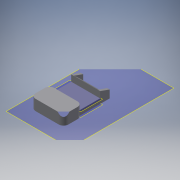
# Autodesk Inventor part: schnapper
Saved by Autodesk Inventor 2016 (Build 200138000, 138)
## iProperties
Created: 2016-06-09
Part Number: schnapper
Material: Generic
Document SubType Name: Modeling
Designer: Chris
Density: 1 g/cm^3
Appearance: Default
Author: Chris
Autodesk Inventor part; units mm, degrees
ref_plane "YZ Plane" through (0, 0, 0) normal (1, 0, 0) x (0, 1, 0)
ref_plane "XZ Plane" through (0, 0, 0) normal (0, 1, 0) x (-1, 0, 0)
ref_plane "XY Plane" through (0, 0, 0) normal (0, 0, 1) x (1, 0, 0)
ref_plane "Work Plane2" through (0, 5.2982, -18) normal (0, 0, -1) x (-1, 0, 0)
ref_plane "Work Plane4" through (0, -4.9464, -12) normal (0, 0, -1) x (-1, 0, 0)
ref_plane "Work Plane3" through (0, -4.9464, -7) normal (0, 0, -1) x (-1, 0, 0)
sketch "Sketch3" plane through (0, 5.2982, -18) normal (0, 0, -1) x (-1, 0, 0)
  line L0 (13, 53.6093) -> (-13, 53.6093) projected
  arc A0 (-13, 53.6093) -> (-30, 36.6093) centre (-13, 36.6093) ccw projected
  line L1 (-30, 36.6093) -> (-30, -44.3907) projected
  line L2 (-30, -44.3907) -> (30, -44.3907) projected
  line L3 (30, -44.3907) -> (30, 36.6093) projected
  arc A1 (30, 36.6093) -> (13, 53.6093) centre (13, 36.6093) ccw projected
  line L4 (-0.95, 23.6093) -> (-0.95, 40.6093) projected
  line L5 (-0.95, 40.6093) -> (0.95, 40.6093) projected
  line L6 (0.95, 40.6093) -> (0.95, 23.6093) projected
  line L7 (0.95, 23.6093) -> (-0.95, 23.6093) projected
  line L8 (6.55, 40.6093) -> (8.45, 40.6093) projected
  line L9 (8.45, 40.6093) -> (8.45, 23.6093) projected
  line L10 (8.45, 23.6093) -> (6.55, 23.6093) projected
  line L11 (6.55, 23.6093) -> (6.55, 40.6093) projected
  line L12 (-8.45, 40.6093) -> (-6.55, 40.6093) projected
  line L13 (-6.55, 40.6093) -> (-6.55, 23.6093) projected
  line L14 (-6.55, 23.6093) -> (-8.45, 23.6093) projected
  line L15 (-8.45, 23.6093) -> (-8.45, 40.6093) projected
  line L16 (-15.5, -21.0481) -> (-15.5, 10.5093) projected
  line L17 (-15.5, 10.5093) -> (-12, 10.5093) projected
  line L18 (-12, 10.5093) -> (-12, 4.9593) projected
  line L19 (-12, 4.9593) -> (12, 4.9593) projected
  line L20 (12, 4.9593) -> (12, 10.5093) projected
  line L21 (12, 10.5093) -> (15.5, 10.5093) projected
  line L22 (15.5, 10.5093) -> (15.5, -21.0481) projected
  arc A2 (17.5, -25.2907) -> (15.5, -21.0481) centre (12, -25.2907) ccw projected
  line L23 (17.5, -25.2907) -> (17.5, -34.7907) projected
  arc A3 (12, -40.2907) -> (17.5, -34.7907) centre (12, -34.7907) ccw projected
  line L24 (12, -40.2907) -> (-12, -40.2907) projected
  arc A4 (-17.5, -34.7907) -> (-12, -40.2907) centre (-12, -34.7907) ccw projected
  line L25 (-17.5, -34.7907) -> (-17.5, -25.2907) projected
  arc A5 (-15.5, -21.0481) -> (-17.5, -25.2907) centre (-12, -25.2907) ccw projected
  line L26 (-15.5, -0.3907) -> (15.5, -0.3907) projected
  line L27 (-15.5, -21.0481) -> (-15.5, -0.3907) projected
  arc A6 (-12, -19.7907) -> (-15.5, -21.0481) centre (-12, -25.2907) ccw projected
  line L28 (12, -19.7907) -> (-12, -19.7907) projected
  arc A7 (15.5, -21.0481) -> (12, -19.7907) centre (12, -25.2907) ccw projected
  line L29 (15.5, -0.3907) -> (15.5, -21.0481) projected
  arc A8 (-15, -21.2907) -> (-17, -25.2907) centre (-12, -25.2907) ccw
  line L30 (-17, -25.2907) -> (-17, -34.7907)
  arc A9 (-17, -34.7907) -> (-12, -39.7907) centre (-12, -34.7907) ccw
  line L31 (-12, -39.7907) -> (12, -39.7907)
  arc A10 (12, -39.7907) -> (17, -34.7907) centre (12, -34.7907) ccw
  line L32 (17, -34.7907) -> (17, -25.2907)
  arc A11 (17, -25.2907) -> (15, -21.2907) centre (12, -25.2907) ccw
  line L33 (-15, -21.2907) -> (-15, 10.0093)
  line L34 (-15, 10.0093) -> (-12.5, 10.0093)
  line L35 (-12.5, 10.0093) -> (-12.5, 4.4593)
  line L36 (-12.5, 4.4593) -> (12.5, 4.4593)
  line L37 (12.5, 4.4593) -> (12.5, 10.0093)
  line L38 (12.5, 10.0093) -> (15, 10.0093)
  line L39 (15, 10.0093) -> (15, -21.2907)
  point P0 (0, -5.2982)
  dimension "d3" = 0.5
  dimension "d4" = 0.5
  constraints: 20 end point, 8 point on circle, 4 centre point, 12 other
  measures "d3" distance between parallel lines of L25 L30
  measures "d4" distance between parallel lines of L16 L33
extrude "Extrusion1" add sketch "Sketch3" against normal up to surface (5 mm away) from surface at -6 contours L33 L26 L39 A7 L28 A6 | A6 L28 A7 L39 A11 L32 A10 L31 A9 L30 A8 L33 | L33 L34 L35 L36 L37 L38 L39 L26
sketch "Sketch4" plane through (-12.5, 9.7575, -7) normal (0, 0, 1) x (1, 0, 0)
  line L0 (29.5, -39.25) -> (29.5, -29.75) projected
  arc A0 (29.5, -29.75) -> (27.5, -25.75) centre (24.5, -29.75) ccw projected
  line L1 (27.5, -25.75) -> (27.5, 5.55) projected
  line L2 (27.5, 5.55) -> (25, 5.55) projected
  line L3 (25, 5.55) -> (25, 0) projected
  line L4 (25, 0) -> (0, 0) projected
  line L5 (0, 0) -> (0, 5.55) projected
  line L6 (0, 5.55) -> (-2.5, 5.55) projected
  line L7 (-2.5, 5.55) -> (-2.5, -25.75) projected
  arc A1 (-2.5, -25.75) -> (-4.5, -29.75) centre (0.5, -29.75) ccw projected
  line L8 (-4.5, -29.75) -> (-4.5, -39.25) projected
  arc A2 (-4.5, -39.25) -> (0.5, -44.25) centre (0.5, -39.25) ccw projected
  line L9 (0.5, -44.25) -> (24.5, -44.25) projected
  arc A3 (24.5, -44.25) -> (29.5, -39.25) centre (24.5, -39.25) ccw projected
  line L10 (0.5, -24.25) -> (24.5, -24.25) projected
  arc A4 (0.5, -24.25) -> (-3, -25.5074) centre (0.5, -29.75) ccw projected
  arc A5 (28, -25.5074) -> (24.5, -24.25) centre (24.5, -29.75) ccw projected
  arc A6 (27.5, -25.75) -> (24.5, -24.75) centre (24.5, -29.75) ccw
  line L11 (24.5, -24.75) -> (0.5, -24.75)
  arc A7 (0.5, -24.75) -> (-2.5, -25.75) centre (0.5, -29.75) ccw
  point P0 (12.5, -9.7575)
  constraints: 4 point on circle, 2 centre point, 2 end point, 2 other
extrude "Extrusion2" add sketch "Sketch4" along normal blind 6 contours A3 L9 A2 L8 A1 A7 L11 A6 A0 L0
sketch "Sketch5" plane through (0, 0, 0) normal (1, 0, 0) x (0, 1, 0)
  line L0 (9.7575, -7) -> (15.3075, -7) projected
  line L1 (4.9075, -6.5) -> (4.9075, -4) projected
  line L2 (15.8075, -4) -> (15.8075, -18) projected
  line L3 (15.3075, -7) -> (-15.9925, -7) projected
  line L4 (4.9075, -4) -> (15.8075, -4) projected
  line L5 (5.4075, -0.5) -> (5.4075, -7)
  line L6 (5.4075, -0.5) -> (15.3075, -4)
  line L7 (15.3075, -4) -> (15.3075, -7)
  point P0 (0, 0)
  dimension "d10" = 0.5
  dimension "d11" = 3.5
  constraints: 6 end point, 2 perpendicular, 2 point on line
  measures "d10" distance between parallel lines of L1 L5
  measures "d11" distance from line of L5.start L4
extrude "Extrusion3" add sketch "Sketch5" against normal up to surface (2.5 mm away) from surface at 15
mirror "Mirror1" about plane through (0, 0, 0) normal (1, 0, 0) of "Extrusion3"
sketch "Sketch6" plane through (0, 0, 0) normal (1, 0, 0) x (0, 1, 0)
  line L0 (5.4075, -7) -> (9.7575, -7) projected
  line L1 (5.4075, -0.5) -> (5.4075, -7) projected
  line L2 (5.4075, -0.5) -> (9.7575, -4)
  line L3 (9.7575, -4) -> (9.7575, -7)
  point P0 (0, 0)
  point P1 (15.3075, -4)
  constraints: 4 end point, 1 horizontal alignment, 1 perpendicular
extrude "Extrusion4" add sketch "Sketch6" along normal up to surface (25 mm away) from surface at -12.5
body "Solid1"
